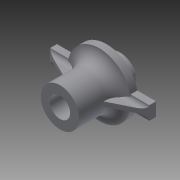
# Autodesk Inventor part: propeller-holder-big
Saved by Autodesk Inventor 2014 SP2 (Build 180247200, 247)
## iProperties
Created: 2016-10-04
Part Number: propeller-holder-big
Material: 一般
Document SubType Name: Modeling
Designer: hide
Density: 1 g/cm^3
Appearance: 既定
Author: hide
Autodesk Inventor part; units mm, degrees
ref_plane "YZ Plane" through (0, 0, 0) normal (1, 0, 0) x (0, 1, 0)
ref_plane "XZ Plane" through (0, 0, 0) normal (0, 1, 0) x (-1, 0, 0)
ref_plane "XY Plane" through (0, 0, 0) normal (0, 0, 1) x (1, 0, 0)
sketch "スケッチ2" plane through (0, 0, 0) normal (0, 1, 0) x (-1, 0, 0)
  circle A0 centre (0, 0) radius 2.25
  circle A1 centre (0, 0) radius 4.25
  dimension "d5" = 2
  dimension "d6" = 4.5
  constraints: 2 centre point, 2 coincident
  measures "d5" radial gap between concentric circles of A0 A1
  measures "d6" diameter of A0
extrude "押し出し1" add sketch "スケッチ2" along normal blind 10.3
sketch "スケッチ3" plane through (0, 0, 0) normal (1, 0, 0) x (0, 1, 0)
  circle A0 centre (3.8, 0) radius 0.75
  point P0 (0, 0)
  dimension "d9" = 1.5
  dimension "d10" = 0
  dimension "d11" = 3.8
  constraints: 1 centre point
  measures "d9" diameter of A0
  measures "d10" vertical distance of point (0, 0) A0.centre
  measures "d11" distance of point (0, 0) A0.centre
extrude "押し出し2" cut sketch "スケッチ3" against normal blind 9.3
sketch "スケッチ4" plane through (0, 10.3, 0) normal (0, 1, 0) x (1, 0, 0)
  circle A0 centre (0, 0) radius 2.25 projected
  circle A1 centre (0, 0) radius 4.25 projected
  line L0 (-7, 7) -> (7, 7)
  line L1 (7, 7) -> (7, -7)
  line L2 (7, -7) -> (-7, -7)
  line L3 (-7, -7) -> (-7, 7)
  dimension "d19" = 14
  dimension "d20" = 7
  dimension "d22" = 14
  dimension "d23" = 7
  constraints: 8 end point, 2 parallel, 1 horizontal, 1 perpendicular
  measures "d19" distance of L2.end L0.start
  measures "d20" distance from line of A0.centre L0
  measures "d22" distance between parallel lines of L3 L1
  measures "d23" distance from line of A0.centre L3
extrude "押し出し3" add sketch "スケッチ4" against normal blind 1.6 contours L0 L1 L2 L3
fillet "フィレット4" radius 7 4 edges at (7, 9.5, 7) (7, 9.5, -7) (-7, 9.5, 7) (-7, 9.5, -7)
sketch "スケッチ9" plane through (0, 10.3, 0) normal (0, 1, 0) x (1, 0, 0)
  circle A0 centre (0, 0) radius 7 projected
  line L0 (-5, 1.5) -> (-11, 1.5)
  line L1 (-11, 1.5) -> (-11, -1.5)
  line L2 (-11, -1.5) -> (-5, -1.5)
  line L3 (-5, -1.5) -> (-5, 1.5)
  dimension "d56" = 5
  dimension "d57" = 6
  dimension "d63" = 3
  dimension "d64" = 1.5
  constraints: 8 end point, 2 parallel, 1 horizontal, 1 perpendicular
  measures "d56" distance from line of A0.centre L3
  measures "d57" distance of L0.start L0.end
  measures "d63" distance of L0.end L1.end
  measures "d64" distance from line of A0.centre L0
extrude "押し出し8" add sketch "スケッチ9" against normal blind 1.5 contours L0 L3 L2 A0 | A0 L2 L1 L0 picked at (-5.6606, 0.1678)
mirror "ミラー1" about plane through (0, 0, 0) normal (1, 0, 0) of "押し出し8"
sketch "スケッチ13" plane through (0, 0, 0) normal (0, 0, 1) x (1, 0, 0)
  line L0 (-6.8374, 10.3) -> (-6.8374, 8.8) projected
  line L1 (-11, 10.3) -> (-6.8374, 10.3) projected
  line L2 (-11, 10.3) -> (-11, 8.8) projected
  line L3 (-6.8374, 8.8) -> (-11, 8.8) projected
  line L4 (-11, 8.8) -> (-3.9094, 5.325)
  line L5 (-3.9094, 5.325) -> (-3.9094, 8.8)
  line L6 (-3.9094, 8.8) -> (-11, 8.8)
  point P0 (0, 0)
  constraints: 6 end point, 2 perpendicular
extrude "押し出し12" add sketch "スケッチ13" along normal mid plane 1 contours L6 L5 L4 L3
mirror "ミラー2" about plane through (0, 0, 0) normal (1, 0, 0) of "押し出し12"
fillet "フィレット5" radius 1 4 edges at (-8.9911, 8.8, -0.5) (-8.9911, 8.8, 0.5) (8.9911, 8.8, 0.5) (8.9911, 8.8, -0.5)
fillet "フィレット6" radius 2.8 2 edges at (0, 8.7, -4.25) (0, 8.7, 4.25)
sketch "スケッチ15" plane through (0, 10.3, 0) normal (0, 1, 0) x (1, 0, 0)
  circle A0 centre (0, 0) radius 2.25 projected
  circle A1 centre (0, 0) radius 3.9
  dimension "d81" = 7.8
  constraints: 1 centre point, 1 coincident
  measures "d81" diameter of A1
extrude "押し出し14" add sketch "スケッチ15" along normal blind 1.5
sketch "スケッチ16" plane through (0, 11.8, 0) normal (0, 1, 0) x (1, 0, 0)
  circle A0 centre (0, 0) radius 2.25 projected
  circle A1 centre (0, 0) radius 3.9 projected
  line L0 (-3.5, 6.3728) -> (3.5, 6.3728)
  line L1 (3.5, 1.7205) -> (3.5, -1.7205)
  line L2 (3.5, -6.211) -> (-3.5, -6.211)
  line L3 (-3.5, -1.7205) -> (-3.5, 1.7205)
  dimension "d84" = 7
  dimension "d85" = 3.5
  constraints: 8 end point, 4 point on circle, 2 parallel, 1 horizontal, 1 perpendicular
  measures "d84" distance of L0.start L0.end
  measures "d85" distance from line of A0.centre L3
extrude "押し出し15" add sketch "スケッチ16" along normal blind 1.5 contours A0 | L1 A1 L3
equation "\"d20\" = 0.5 * d19"
equation "\"d22\" = d19"
equation "\"d23\" = 0.5 * d22"
equation "\"d64\" = 0.5 * d63"
equation "\"d85\" = 0.5 * d84"
